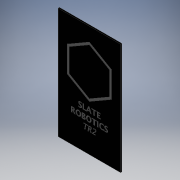
# Autodesk Inventor part: BA03
Saved by Autodesk Inventor 2017 (Build 210142000, 142)
## iProperties
Created: 2018-10-18
Part Number: BA03
Material: ABS Plastic
Document SubType Name: Modeling
Designer: Dell
Density: 1.06 g/cm^3
Appearance: Smooth - Black
Author: Dell
Autodesk Inventor part; units mm, degrees
ref_plane "YZ Plane" through (0, 0, 0) normal (1, 0, 0) x (0, 1, 0)
ref_plane "XZ Plane" through (0, 0, 0) normal (0, 1, 0) x (-1, 0, 0)
ref_plane "XY Plane" through (0, 0, 0) normal (0, 0, 1) x (1, 0, 0)
sketch "Sketch1" plane through (0, 0, 0) normal (0, 0, 1) x (1, 0, 0)
  line L0 (0, 0) -> (303.5592, 0)
  line L1 (303.5592, 0) -> (303.5592, -533.4)
  line L2 (303.5592, -533.4) -> (0, -533.4)
  line L3 (0, -533.4) -> (0, 0)
  line L4 (455.3388, 262.89) -> (303.5592, 0)
  line L5 (303.5592, 0) -> (0, 0)
  line L6 (0, 0) -> (-151.7796, 262.89)
  line L7 (-151.7796, 262.89) -> (0, 525.78)
  line L8 (0, 525.78) -> (303.5592, 525.78)
  line L9 (303.5592, 525.78) -> (455.3388, 262.89)
  point P0 (151.7796, 262.89)
  dimension "d1" = 533.4
  dimension "d76" = 525.78
  constraints: 20 end point, 2 parallel, 1 horizontal, 1 perpendicular, 13 other
  measures "d1" distance of L0.end L1.end
  measures "d76" distance between parallel lines of L4 L7
extrude "Extrusion1" add sketch "Sketch1" along normal blind 6.35 contours L0 L1 L2 L3
sketch "Sketch2" plane through (0, 0, 0) normal (0, 1, 0) x (1, 0, 0)
  line L0 (303.5592, -6.35) -> (0, -6.35) projected
  line L1 (0, -6.35) -> (-3.6662, -6.35)
  line L2 (-3.6662, -6.35) -> (0, 0)
  line L3 (0, 0) -> (0, -6.35) projected
  line L4 (0, 0) -> (0, -6.35) projected
  line L5 (0, -6.35) -> (0, 0)
  line L6 (303.5592, -6.35) -> (307.2254, -6.35)
  line L7 (303.5592, 0) -> (303.5592, -6.35) projected
  line L8 (307.2254, -6.35) -> (303.5592, 0)
  line L9 (303.5592, 0) -> (303.5592, -6.35)
  dimension "d4" = 30
  dimension "d5" = 60
  constraints: 12 end point, 2 collinear, 2 horizontal
  measures "d4" angle of L3 L2
  measures "d5" angle of L6 L8
extrude "Extrusion2" add sketch "Sketch2" against normal blind 533.4
sketch "Sketch6" plane through (0, 0, 6.35) normal (0, 0, 1) x (1, 0, 0)
  line L0 (26.7796, -316.7) -> (276.7796, -316.7) construction
  line L1 (276.7796, -316.7) -> (276.7796, -466.7) construction
  line L2 (276.7796, -466.7) -> (26.7796, -466.7) construction
  line L3 (26.7796, -466.7) -> (26.7796, -316.7) construction
  line L4 (26.7796, -66.7) -> (276.7796, -66.7) construction
  line L5 (276.7796, -66.7) -> (276.7796, -316.7) construction
  line L6 (276.7796, -316.7) -> (26.7796, -316.7) construction
  line L7 (26.7796, -316.7) -> (26.7796, -66.7) construction
  line L8 (276.7796, -466.7) -> (276.7796, -66.7) construction
  line L9 (151.7796, -66.7) -> (260.0328, -129.2)
  line L10 (260.0328, -129.2) -> (260.0328, -254.2)
  line L11 (260.0328, -254.2) -> (151.7796, -316.7)
  line L12 (151.7796, -316.7) -> (43.5264, -254.2)
  line L13 (43.5264, -254.2) -> (43.5264, -129.2)
  line L14 (43.5264, -129.2) -> (151.7796, -66.7)
  line L15 (151.7796, -78.4779) -> (249.8328, -135.089)
  line L16 (249.8328, -135.089) -> (249.8328, -248.311)
  line L17 (249.8328, -248.311) -> (151.7796, -304.9221)
  line L18 (151.7796, -304.9221) -> (53.7264, -248.311)
  line L19 (53.7264, -248.311) -> (53.7264, -135.089)
  line L20 (53.7264, -135.089) -> (151.7796, -78.4779)
  line L21 (151.7796, -83.3854) -> (245.5828, -137.5427) construction
  line L22 (245.5828, -137.5427) -> (245.5828, -245.8573)
  line L23 (245.5828, -245.8573) -> (151.7796, -300.0146)
  line L24 (151.7796, -300.0146) -> (57.9764, -245.8573)
  line L25 (57.9764, -245.8573) -> (57.9764, -137.5427)
  line L26 (57.9764, -137.5427) -> (151.7796, -83.3854) construction
  line L27 (57.9764, -190.0427) -> (97.9764, -166.9487)
  line L28 (97.9764, -166.9487) -> (97.9764, -138.4487)
  line L29 (97.9764, -138.4487) -> (111.9764, -138.4487)
  line L30 (111.9764, -138.4487) -> (111.9764, -158.8658)
  line L31 (111.9764, -158.8658) -> (151.7796, -135.8854)
  line L32 (151.7796, -135.8854) -> (245.5828, -190.0427)
  line L33 (245.5828, -190.0427) -> (245.5828, -137.5427)
  line L34 (245.5828, -137.5427) -> (151.7796, -83.3854)
  line L35 (151.7796, -83.3854) -> (57.9764, -137.5427)
  line L36 (57.9764, -190.0427) -> (57.9764, -137.5427)
  line L37 (57.9764, -245.8573) -> (139.7796, -293.0864)
  line L38 (139.7796, -293.0864) -> (139.7796, -253.0146)
  line L39 (139.7796, -253.0146) -> (163.7796, -253.0146)
  line L40 (163.7796, -253.0146) -> (163.7796, -293.0864)
  line L41 (163.7796, -293.0864) -> (245.5828, -245.8573)
  line L42 (245.5828, -245.8573) -> (245.5828, -205.0427)
  line L43 (245.5828, -205.0427) -> (151.7796, -150.8854)
  line L44 (151.7796, -150.8854) -> (57.9764, -205.0427)
  line L45 (57.9764, -205.0427) -> (57.9764, -245.8573)
  line L46 (125.5296, -179.0146) -> (178.0296, -179.0146) construction
  line L47 (178.0296, -179.0146) -> (178.0296, -230.0146) construction
  line L48 (178.0296, -230.0146) -> (125.5296, -230.0146) construction
  line L49 (125.5296, -230.0146) -> (125.5296, -179.0146) construction
  line L50 (125.5296, -230.0146) -> (149.5296, -230.0146)
  line L51 (149.5296, -230.0146) -> (149.5296, -206.0146)
  line L52 (149.5296, -206.0146) -> (125.5296, -206.0146)
  line L53 (125.5296, -206.0146) -> (125.5296, -230.0146)
  line L54 (125.5296, -179.0146) -> (149.5296, -179.0146)
  line L55 (149.5296, -179.0146) -> (149.5296, -203.0146)
  line L56 (149.5296, -203.0146) -> (125.5296, -203.0146)
  line L57 (125.5296, -203.0146) -> (125.5296, -179.0146)
  line L58 (178.0296, -179.0146) -> (154.0296, -179.0146)
  line L59 (154.0296, -179.0146) -> (154.0296, -203.0146)
  line L60 (154.0296, -203.0146) -> (178.0296, -203.0146)
  line L61 (178.0296, -203.0146) -> (178.0296, -179.0146)
  line L62 (178.0296, -230.0146) -> (154.0296, -230.0146)
  line L63 (154.0296, -230.0146) -> (154.0296, -206.0146)
  line L64 (154.0296, -206.0146) -> (178.0296, -206.0146)
  line L65 (178.0296, -206.0146) -> (178.0296, -230.0146)
  line L66 (-3.6662, 0) -> (307.2254, 0) projected
  line L67 (-3.6662, 0) -> (-3.6662, -533.4) projected
  line L68 (98.5279, -364.3042) -> (98.5279, -360.0196)
  spline S0 degree 2 poles (98.5279, -360.0196) (101.4544, -361.2437) (104.3427, -361.7219) (105.5478, -361.7219) knots 0 0 0 1 2 2 2
  spline S1 degree 2 poles (105.5478, -361.7219) (107.7284, -361.7219) (109.8898, -359.7709) (109.8898, -358.3937) knots 0 0 0 1 2 2 2
  spline S2 degree 2 poles (109.8898, -358.3937) (109.8898, -357.3417) (109.2968, -356.5) knots 0 0 0 1 1 1
  spline S3 degree 2 poles (109.2968, -356.5) (108.6847, -355.6776) (106.332, -354.3577) knots 0 0 0 1 1 1
  line L69 (106.332, -354.3577) -> (104.6488, -353.4205)
  spline S4 degree 2 poles (104.6488, -353.4205) (101.0336, -351.4121) (99.7712, -349.7097) knots 0 0 0 1 1 1
  spline S5 degree 2 poles (99.7712, -349.7097) (98.4705, -348.0073) (98.4705, -345.7694) knots 0 0 0 1 1 1
  spline S6 degree 2 poles (98.4705, -345.7694) (98.4705, -342.9385) (102.7934, -338.9216) (106.8293, -338.9216) knots 0 0 0 1 2 2 2
  spline S7 degree 2 poles (106.8293, -338.9216) (109.8515, -338.9216) (113.6388, -339.7824) knots 0 0 0 1 1 1
  line L70 (113.6388, -339.7824) -> (113.6388, -343.7801)
  spline S8 degree 2 poles (113.6388, -343.7801) (109.7559, -342.3455) (107.4797, -342.3455) knots 0 0 0 1 1 1
  spline S9 degree 2 poles (107.4797, -342.3455) (105.586, -342.3455) (103.6159, -343.9905) (103.6159, -345.1382) knots 0 0 0 1 2 2 2
  spline S10 degree 2 poles (103.6159, -345.1382) (103.6159, -346.018) (104.228, -346.764) knots 0 0 0 1 1 1
  spline S11 degree 2 poles (104.228, -346.764) (104.8018, -347.5291) (107.1545, -348.8489) knots 0 0 0 1 1 1
  line L71 (107.1545, -348.8489) -> (108.9525, -349.8436)
  spline S12 degree 2 poles (108.9525, -349.8436) (113.1033, -352.158) (114.2318, -353.8604) knots 0 0 0 1 1 1
  spline S13 degree 2 poles (114.2318, -353.8604) (115.3603, -355.5819) (115.3603, -357.7242) knots 0 0 0 1 1 1
  spline S14 degree 2 poles (115.3603, -357.7242) (115.3603, -360.8038) (110.674, -365.1458) (105.5669, -365.1458) knots 0 0 0 1 2 2 2
  spline S15 degree 2 poles (105.5669, -365.1458) (102.5447, -365.1458) (98.5279, -364.3042) knots 0 0 0 1 1 1
  line L72 (119.6832, -364.5337) -> (119.6832, -339.5337)
  line L73 (119.6832, -339.5337) -> (124.886, -339.5337)
  line L74 (124.886, -339.5337) -> (124.886, -360.9951)
  line L75 (124.886, -360.9951) -> (136.0375, -360.9951)
  line L76 (136.0375, -360.9951) -> (136.0375, -364.5337)
  line L77 (136.0375, -364.5337) -> (119.6832, -364.5337)
  line L78 (137.0512, -364.5337) -> (146.749, -339.5337)
  line L79 (146.749, -339.5337) -> (151.9709, -339.5337)
  line L80 (151.9709, -339.5337) -> (161.7069, -364.5337)
  line L81 (161.7069, -364.5337) -> (156.3703, -364.5337)
  line L82 (156.3703, -364.5337) -> (153.7689, -357.8581)
  line L83 (153.7689, -357.8581) -> (143.4399, -357.8581)
  line L84 (143.4399, -357.8581) -> (140.8385, -364.5337)
  line L85 (140.8385, -364.5337) -> (137.0512, -364.5337)
  line L86 (144.7215, -354.5299) -> (152.4682, -354.5299)
  line L87 (152.4682, -354.5299) -> (148.6044, -344.5643)
  line L88 (148.6044, -344.5643) -> (144.7215, -354.5299)
  line L89 (171.4621, -364.5337) -> (171.4621, -342.9767)
  line L90 (171.4621, -342.9767) -> (162.5103, -342.9767)
  line L91 (162.5103, -342.9767) -> (162.5103, -339.5337)
  line L92 (162.5103, -339.5337) -> (185.6166, -339.5337)
  line L93 (185.6166, -339.5337) -> (185.6166, -342.9767)
  line L94 (185.6166, -342.9767) -> (176.6648, -342.9767)
  line L95 (176.6648, -342.9767) -> (176.6648, -364.5337)
  line L96 (176.6648, -364.5337) -> (171.4621, -364.5337)
  line L97 (189.0979, -364.5337) -> (189.0979, -339.5337)
  line L98 (189.0979, -339.5337) -> (205.1078, -339.5337)
  line L99 (205.1078, -339.5337) -> (205.1078, -342.9767)
  line L100 (205.1078, -342.9767) -> (194.3007, -342.9767)
  line L101 (194.3007, -342.9767) -> (194.3007, -349.9392)
  line L102 (194.3007, -349.9392) -> (203.2333, -349.9392)
  line L103 (203.2333, -349.9392) -> (203.2333, -353.3822)
  line L104 (203.2333, -353.3822) -> (194.3007, -353.3822)
  line L105 (194.3007, -353.3822) -> (194.3007, -360.9951)
  line L106 (194.3007, -360.9951) -> (205.9112, -360.9951)
  line L107 (205.9112, -360.9951) -> (205.9112, -364.5337)
  line L108 (205.9112, -364.5337) -> (189.0979, -364.5337)
  line L109 (63.7632, -404.4902) -> (63.7632, -379.4902)
  line L110 (63.7632, -379.4902) -> (73.1166, -379.4902)
  spline S16 degree 2 poles (73.1166, -379.4902) (75.9858, -379.4902) (78.9889, -380.9248) (80.7295, -383.8514) (80.7295, -385.6876) knots 0 0 0 1 2 3 3 3
  spline S17 degree 2 poles (80.7295, -385.6876) (80.7295, -387.8873) (78.2046, -391.7894) (75.8902, -392.8223) knots 0 0 0 1 2 2 2
  line L111 (75.8902, -392.8223) -> (84.0577, -404.4902)
  line L112 (84.0577, -404.4902) -> (77.7264, -404.4902)
  line L113 (77.7264, -404.4902) -> (71.5099, -394.276)
  line L114 (71.5099, -394.276) -> (68.6599, -394.276)
  line L115 (68.6599, -394.276) -> (68.6599, -404.4902)
  line L116 (68.6599, -404.4902) -> (63.7632, -404.4902)
  line L117 (68.6599, -390.8521) -> (69.8458, -390.8521)
  spline S18 degree 2 poles (69.8458, -390.8521) (73.0593, -390.8521) (75.5267, -388.0403) (75.5267, -386.2615) knots 0 0 0 1 2 2 2
  spline S19 degree 2 poles (75.5267, -386.2615) (75.5267, -384.7312) (73.5375, -382.9141) (70.477, -382.9141) knots 0 0 0 1 2 2 2
  line L118 (70.477, -382.9141) -> (68.6599, -382.9141)
  line L119 (68.6599, -382.9141) -> (68.6599, -390.8521)
  spline S20 degree 2 poles (98.7479, -405.1023) (94.8458, -405.1023) (89.0692, -401.8697) (86.0662, -395.8253) (86.0662, -391.9807) knots 0 0 0 1 2 3 3 3
  spline S21 degree 2 poles (86.0662, -391.9807) (86.0662, -388.1742) (89.0692, -382.0916) (94.8841, -378.8781) (98.7479, -378.8781) knots 0 0 0 1 2 3 3 3
  spline S22 degree 2 poles (98.7479, -378.8781) (102.5925, -378.8781) (108.4074, -382.0916) (111.4105, -388.1742) (111.4105, -391.9807) knots 0 0 0 1 2 3 3 3
  spline S23 degree 2 poles (111.4105, -391.9807) (111.4105, -395.8253) (108.4074, -401.8697) (102.6499, -405.1023) (98.7479, -405.1023) knots 0 0 0 1 2 3 3 3
  spline S24 degree 2 poles (98.7479, -401.6784) (102.363, -401.6784) (105.8825, -395.7871) (105.8825, -391.9807) knots 0 0 0 1 2 2 2
  spline S25 degree 2 poles (105.8825, -391.9807) (105.8825, -388.1551) (102.3439, -382.302) (98.7479, -382.302) knots 0 0 0 1 2 2 2
  spline S26 degree 2 poles (98.7479, -382.302) (95.1327, -382.302) (91.5941, -388.1551) (91.5941, -391.9807) knots 0 0 0 1 2 2 2
  spline S27 degree 2 poles (91.5941, -391.9807) (91.5941, -395.7871) (95.1136, -401.6784) (98.7479, -401.6784) knots 0 0 0 1 2 2 2
  line L120 (116.0776, -404.4902) -> (116.0776, -379.4902)
  line L121 (116.0776, -379.4902) -> (124.513, -379.4902)
  spline S28 degree 2 poles (124.513, -379.4902) (127.5734, -379.4902) (130.5, -380.8674) (132.1641, -383.5453) (132.1641, -385.0564) knots 0 0 0 1 2 3 3 3
  spline S29 degree 2 poles (132.1641, -385.0564) (132.1641, -386.9309) (129.5627, -390.3739) (126.1962, -391.426) knots 0 0 0 1 2 2 2
  spline S30 degree 2 poles (126.1962, -391.426) (128.8741, -392.0954) (131.705, -394.0465) (133.1779, -396.7626) (133.1779, -398.312) knots 0 0 0 1 2 3 3 3
  spline S31 degree 2 poles (133.1779, -398.312) (133.1779, -399.9952) (131.4564, -402.9217) (128.4342, -404.4902) (125.2972, -404.4902) knots 0 0 0 1 2 3 3 3
  line L122 (125.2972, -404.4902) -> (116.0776, -404.4902)
  line L123 (121.07, -400.9516) -> (122.0646, -400.9516)
  spline S32 degree 2 poles (122.0646, -400.9516) (124.7808, -400.9516) (126.7509, -400.2439) (127.7456, -398.6563) (127.7456, -397.6807) knots 0 0 0 1 2 3 3 3
  spline S33 degree 2 poles (127.7456, -397.6807) (127.7456, -395.8253) (124.4747, -393.2431) (121.969, -393.2431) knots 0 0 0 1 2 2 2
  line L124 (121.969, -393.2431) -> (121.07, -393.2431)
  line L125 (121.07, -393.2431) -> (121.07, -400.9516)
  line L126 (121.07, -389.8957) -> (122.1794, -389.8957)
  spline S34 degree 2 poles (122.1794, -389.8957) (124.5512, -389.8957) (126.8848, -387.543) (126.8848, -385.8598) knots 0 0 0 1 2 2 2
  spline S35 degree 2 poles (126.8848, -385.8598) (126.8848, -384.9608) (126.1962, -383.6409) (124.4556, -382.9141) (122.0072, -382.9141) knots 0 0 0 1 2 3 3 3
  line L127 (122.0072, -382.9141) -> (121.07, -382.9141)
  line L128 (121.07, -382.9141) -> (121.07, -389.8957)
  spline S36 degree 2 poles (148.9965, -405.1023) (145.0945, -405.1023) (139.3179, -401.8697) (136.3148, -395.8253) (136.3148, -391.9807) knots 0 0 0 1 2 3 3 3
  spline S37 degree 2 poles (136.3148, -391.9807) (136.3148, -388.1742) (139.3179, -382.0916) (145.1327, -378.8781) (148.9965, -378.8781) knots 0 0 0 1 2 3 3 3
  spline S38 degree 2 poles (148.9965, -378.8781) (152.8412, -378.8781) (158.6561, -382.0916) (161.6591, -388.1742) (161.6591, -391.9807) knots 0 0 0 1 2 3 3 3
  spline S39 degree 2 poles (161.6591, -391.9807) (161.6591, -395.8253) (158.6561, -401.8697) (152.8986, -405.1023) (148.9965, -405.1023) knots 0 0 0 1 2 3 3 3
  spline S40 degree 2 poles (148.9965, -401.6784) (152.6117, -401.6784) (156.1312, -395.7871) (156.1312, -391.9807) knots 0 0 0 1 2 2 2
  spline S41 degree 2 poles (156.1312, -391.9807) (156.1312, -388.1551) (152.5925, -382.302) (148.9965, -382.302) knots 0 0 0 1 2 2 2
  spline S42 degree 2 poles (148.9965, -382.302) (145.3814, -382.302) (141.8427, -388.1551) (141.8427, -391.9807) knots 0 0 0 1 2 2 2
  spline S43 degree 2 poles (141.8427, -391.9807) (141.8427, -395.7871) (145.3622, -401.6784) (148.9965, -401.6784) knots 0 0 0 1 2 2 2
  line L129 (172.5428, -404.4902) -> (172.5428, -382.9332)
  line L130 (172.5428, -382.9332) -> (163.591, -382.9332)
  line L131 (163.591, -382.9332) -> (163.591, -379.4902)
  line L132 (163.591, -379.4902) -> (186.6974, -379.4902)
  line L133 (186.6974, -379.4902) -> (186.6974, -382.9332)
  line L134 (186.6974, -382.9332) -> (177.7456, -382.9332)
  line L135 (177.7456, -382.9332) -> (177.7456, -404.4902)
  line L136 (177.7456, -404.4902) -> (172.5428, -404.4902)
  line L137 (190.1786, -404.4902) -> (190.1786, -379.4902)
  line L138 (190.1786, -379.4902) -> (195.3814, -379.4902)
  line L139 (195.3814, -379.4902) -> (195.3814, -404.4902)
  line L140 (195.3814, -404.4902) -> (190.1786, -404.4902)
  spline S44 degree 2 poles (221.7586, -403.4956) (220.1136, -404.2224) (217.6844, -404.758) (214.6048, -405.1023) (213.0937, -405.1023) knots 0 0 0 1 2 3 3 3
  spline S45 degree 2 poles (213.0937, -405.1023) (206.5329, -405.1023) (200.0868, -397.719) (200.0868, -391.9807) knots 0 0 0 1 2 2 2
  spline S46 degree 2 poles (200.0868, -391.9807) (200.0868, -386.2423) (206.5137, -378.8781) (213.4189, -378.8781) knots 0 0 0 1 2 2 2
  spline S47 degree 2 poles (213.4189, -378.8781) (217.4931, -378.8781) (221.529, -379.8345) knots 0 0 0 1 1 1
  line L141 (221.529, -379.8345) -> (221.529, -383.9087)
  spline S48 degree 2 poles (221.529, -383.9087) (219.578, -383.2393) (217.1105, -382.608) (214.9108, -382.302) (213.8014, -382.302) knots 0 0 0 1 2 3 3 3
  spline S49 degree 2 poles (213.8014, -382.302) (209.4977, -382.302) (205.6147, -387.8299) (205.6147, -391.9233) knots 0 0 0 1 2 2 2
  spline S50 degree 2 poles (205.6147, -391.9233) (205.6147, -396.2079) (210.0141, -401.5063) (214.3753, -401.5063) knots 0 0 0 1 2 2 2
  spline S51 degree 2 poles (214.3753, -401.5063) (218.0095, -401.5063) (221.7586, -399.67) knots 0 0 0 1 1 1
  line L142 (221.7586, -399.67) -> (221.7586, -403.4956)
  line L143 (224.8764, -404.2607) -> (224.8764, -399.9761)
  spline S52 degree 2 poles (224.8764, -399.9761) (227.803, -401.2002) (230.6912, -401.6784) (231.8963, -401.6784) knots 0 0 0 1 2 2 2
  spline S53 degree 2 poles (231.8963, -401.6784) (234.0769, -401.6784) (236.2383, -399.7274) (236.2383, -398.3502) knots 0 0 0 1 2 2 2
  spline S54 degree 2 poles (236.2383, -398.3502) (236.2383, -397.2982) (235.6453, -396.4566) knots 0 0 0 1 1 1
  spline S55 degree 2 poles (235.6453, -396.4566) (235.0333, -395.6341) (232.6805, -394.3142) knots 0 0 0 1 1 1
  line L144 (232.6805, -394.3142) -> (230.9973, -393.377)
  spline S56 degree 2 poles (230.9973, -393.377) (227.3821, -391.3686) (226.1197, -389.6662) knots 0 0 0 1 1 1
  spline S57 degree 2 poles (226.1197, -389.6662) (224.819, -387.9638) (224.819, -385.7259) knots 0 0 0 1 1 1
  spline S58 degree 2 poles (224.819, -385.7259) (224.819, -382.895) (229.1419, -378.8781) (233.1779, -378.8781) knots 0 0 0 1 2 2 2
  spline S59 degree 2 poles (233.1779, -378.8781) (236.2, -378.8781) (239.9873, -379.7389) knots 0 0 0 1 1 1
  line L145 (239.9873, -379.7389) -> (239.9873, -383.7366)
  spline S60 degree 2 poles (239.9873, -383.7366) (236.1044, -382.302) (233.8282, -382.302) knots 0 0 0 1 1 1
  spline S61 degree 2 poles (233.8282, -382.302) (231.9346, -382.302) (229.9644, -383.947) (229.9644, -385.0947) knots 0 0 0 1 2 2 2
  spline S62 degree 2 poles (229.9644, -385.0947) (229.9644, -385.9745) (230.5765, -386.7205) knots 0 0 0 1 1 1
  spline S63 degree 2 poles (230.5765, -386.7205) (231.1503, -387.4856) (233.503, -388.8054) knots 0 0 0 1 1 1
  line L146 (233.503, -388.8054) -> (235.301, -389.8001)
  spline S64 degree 2 poles (235.301, -389.8001) (239.4518, -392.1146) (240.5803, -393.8169) knots 0 0 0 1 1 1
  spline S65 degree 2 poles (240.5803, -393.8169) (241.7088, -395.5384) (241.7088, -397.6807) knots 0 0 0 1 1 1
  spline S66 degree 2 poles (241.7088, -397.6807) (241.7088, -400.7603) (237.0225, -405.1023) (231.9154, -405.1023) knots 0 0 0 1 2 2 2
  spline S67 degree 2 poles (231.9154, -405.1023) (228.8932, -405.1023) (224.8764, -404.2607) knots 0 0 0 1 1 1
  line L147 (128.1258, -444.4784) -> (132.5873, -422.1322)
  line L148 (132.5873, -422.1322) -> (123.7027, -422.1322)
  line L149 (123.7027, -422.1322) -> (124.2219, -419.4784)
  line L150 (124.2219, -419.4784) -> (145.5104, -419.4784)
  line L151 (145.5104, -419.4784) -> (144.9719, -422.1322)
  line L152 (144.9719, -422.1322) -> (136.1065, -422.1322)
  line L153 (136.1065, -422.1322) -> (131.6642, -444.4784)
  line L154 (131.6642, -444.4784) -> (128.1258, -444.4784)
  line L155 (143.9142, -444.4784) -> (148.895, -419.4784)
  line L156 (148.895, -419.4784) -> (156.4335, -419.4784)
  spline S68 degree 2 poles (156.4335, -419.4784) (158.4142, -419.4784) (161.1258, -420.1515) (162.9142, -422.5745) (162.9142, -424.3245) knots 0 0 0 1 2 3 3 3
  spline S69 degree 2 poles (162.9142, -424.3245) (162.9142, -426.863) (159.2988, -431.363) (156.2219, -432.5361) knots 0 0 0 1 2 2 2
  line L157 (156.2219, -432.5361) -> (162.1642, -444.4784)
  line L158 (162.1642, -444.4784) -> (158.2412, -444.4784)
  line L159 (158.2412, -444.4784) -> (152.9912, -433.4207)
  line L160 (152.9912, -433.4207) -> (149.645, -433.4207)
  line L161 (149.645, -433.4207) -> (147.4527, -444.4784)
  line L162 (147.4527, -444.4784) -> (143.9142, -444.4784)
  line L163 (150.1642, -430.8053) -> (152.1258, -430.8053)
  spline S70 degree 2 poles (152.1258, -430.8053) (154.2219, -430.8053) (157.3181, -429.2284) (159.145, -426.2284) (159.145, -424.7284) knots 0 0 0 1 2 3 3 3
  spline S71 degree 2 poles (159.145, -424.7284) (159.145, -423.4399) (157.1835, -422.1322) (154.145, -422.1322) knots 0 0 0 1 2 2 2
  line L164 (154.145, -422.1322) -> (151.895, -422.1322)
  line L165 (151.895, -422.1322) -> (150.1642, -430.8053)
  line L166 (165.8565, -444.4784) -> (166.395, -441.7861)
  spline S72 degree 2 poles (166.395, -441.7861) (167.5296, -439.7091) (170.7412, -436.4015) (173.0873, -434.5938) knots 0 0 0 1 2 2 2
  line L167 (173.0873, -434.5938) -> (175.1835, -432.9976)
  spline S73 degree 2 poles (175.1835, -432.9976) (178.1642, -430.7091) (179.7604, -428.7668) knots 0 0 0 1 1 1
  spline S74 degree 2 poles (179.7604, -428.7668) (180.5681, -427.7861) (181.3758, -425.8438) (181.3758, -424.8822) knots 0 0 0 1 2 2 2
  spline S75 degree 2 poles (181.3758, -424.8822) (181.3758, -423.3053) (179.2027, -421.363) (177.0681, -421.363) knots 0 0 0 1 2 2 2
  spline S76 degree 2 poles (177.0681, -421.363) (174.0681, -421.363) (170.4719, -423.4015) knots 0 0 0 1 1 1
  line L168 (170.4719, -423.4015) -> (171.0681, -420.4207)
  spline S77 degree 2 poles (171.0681, -420.4207) (171.645, -420.2091) (171.9142, -420.0745) knots 0 0 0 1 1 1
  spline S78 degree 2 poles (171.9142, -420.0745) (175.2027, -418.863) (177.9142, -418.863) knots 0 0 0 1 1 1
  spline S79 degree 2 poles (177.9142, -418.863) (181.1065, -418.863) (184.9142, -421.6515) (184.9142, -424.4784) knots 0 0 0 1 2 2 2
  spline S80 degree 2 poles (184.9142, -424.4784) (184.9142, -425.9784) (184.3758, -427.3053) knots 0 0 0 1 1 1
  spline S81 degree 2 poles (184.3758, -427.3053) (183.5681, -429.3438) (180.6258, -432.1899) (177.9142, -434.1707) knots 0 0 0 1 2 2 2
  line L169 (177.9142, -434.1707) -> (175.8181, -435.6899)
  spline S82 degree 2 poles (175.8181, -435.6899) (173.9335, -437.0745) (172.5296, -438.3822) (171.8758, -439.1707) knots 0 0 0 1 2 2 2
  spline S83 degree 2 poles (171.8758, -439.1707) (171.4912, -439.6707) (170.7796, -440.6322) (170.3758, -441.5745) knots 0 0 0 1 2 2 2
  line L170 (170.3758, -441.5745) -> (181.3373, -441.5745)
  line L171 (181.3373, -441.5745) -> (180.7412, -444.4784)
  line L172 (180.7412, -444.4784) -> (165.8565, -444.4784)
  point P0 (0, 0)
  point P1 (151.7796, -191.7)
  point P2 (151.7796, -253.0146)
  point P3 (151.7796, -179.0146)
  point P4 (276.7796, -266.7)
  point P5 (-3.6662, -266.7)
  point P6 (151.7796, 0)
  dimension "d27" = 250
  dimension "d28" = 10.2
  dimension "d29" = 4.25
  dimension "d30" = 52.5
  dimension "d31" = 40
  dimension "d32" = 14
  dimension "d33" = 28.5
  dimension "d34" = 15
  dimension "d35" = 24
  dimension "d36" = 47
  dimension "d37" = 23
  dimension "d38" = 51
  dimension "d39" = 52.5
  dimension "d40" = 24
  dimension "d41" = 24
  dimension "d42" = 24
  dimension "d43" = 24
  dimension "d44" = 24
  dimension "d45" = 24
  dimension "d46" = 24
  dimension "d47" = 24
  dimension "d66" = 150
  constraints: 116 end point, 15 parallel, 9 perpendicular, 9 point on line, 8 midpoint, 6 vertical alignment, 5 horizontal, 4 collinear, 2 coincident, 2 vertical, 1 horizontal alignment, 26 other
  measures "d27" distance of L7.end L5.start
  measures "d28" distance between parallel lines of L14 L20
  measures "d29" distance between parallel lines of L20 L26
  measures "d30" distance of L27.start L25.end
  measures "d31" distance between parallel lines of L25 L28
  measures "d32" distance of L28.end L29.end
  measures "d33" distance of L27.end L28.end
  measures "d34" distance of L32.start L43.end
  measures "d35" distance between parallel lines of L40 L38
  measures "d36" distance from line of L24.start L39
  measures "d37" distance between parallel lines of L39 L48
  measures "d38" distance of L50.start L54.start
  measures "d39" distance of L54.start L61.end
  measures "d40" distance of L52.end L52.start
  measures "d41" distance of L52.start L51.start
  measures "d42" distance of L55.end L57.start
  measures "d43" distance of L55.start L55.end
  measures "d44" distance of L61.start L59.end
  measures "d45" distance of L59.end L59.start
  measures "d46" distance of L64.start L64.end
  measures "d47" distance of L63.start L64.start
  measures "d66" distance between parallel lines of L2 L6
extrude "Extrusion5" cut sketch "Sketch6" against normal blind 2 contours L9 L10 L11 L12 L13 L14 | L22 L32 L31 L30 L29 L28 L27 L25 L35 L34 | L22 L43 L44 L25 L27 L28 L29 L30 L31 L32 | L22 L23 L40 L39 L38 L24 L25 L44 L43 | L23 L24 L38 L39 L40 | L53 L52 L51 L50 | L54 L55 L56 L57 | L61 L60 L59 L58 | L62 L63 L64 L65 | L68 S0 S1 S2 S3 L69 S4 S5 S6 S7 L70 S8 S9 S10 S11 L71 S12 S13 S14 S15 | L72 L73 L74 L75 L76 L77 | L78 L79 L80 L81 L82 L83 L84 L85 | L89 L90 L91 L92 L93 L94 L95 L96 | L97 L98 L99 L100 L101 L102 L103 L104 L105 L106 L107 L108 | L109 L110 S16 S17 L111 L112 L113 L114 L115 L116 | S20 S21 S22 S23 | L120 L121 S28 S29 S30 S31 L122 | S36 S37 S38 S39 | L129 L130 L131 L132 L133 L134 L135 L136 | L137 L138 L139 L140 | S44 S45 S46 S47 L141 S48 S49 S50 S51 L142 | L143 S52 S53 S54 S55 L144 S56 S57 S58 S59 L145 S60 S61 S62 S63 L146 S64 S65 S66 S67 | L147 L148 L149 L150 L151 L152 L153 L154 | L155 L156 S68 S69 L157 L158 L159 L160 L161 L162 | L166 S72 L167 S73 S74 S75 S76 L168 S77 S78 S79 S80 S81 L169 S82 S83 L170 L171 L172
extrude "Extrusion6" add sketch "Sketch6" against normal blind 2 contours L22 L32 L31 L30 L29 L28 L27 L25 L35 L34 | L22 L43 L44 L25 L27 L28 L29 L30 L31 L32 | L22 L23 L40 L39 L38 L24 L25 L44 L43 | L23 L24 L38 L39 L40 | L53 L52 L51 L50 | L54 L55 L56 L57 | L61 L60 L59 L58 | L62 L63 L64 L65
sketch "Sketch7" plane through (0, 0, 0) normal (0, 1, 0) x (1, 0, 0)
  line L0 (-3.6662, -6.35) -> (0, 0) projected
  line L1 (0, 0) -> (-3.6662, 0)
  line L2 (-3.6662, 0) -> (-3.6662, -6.35)
  line L3 (-3.6662, -6.35) -> (0, -6.35)
  line L4 (0, -6.35) -> (0, 0)
  line L5 (303.5592, 0) -> (0, 0) projected
  line L6 (303.5592, 0) -> (307.2254, -6.35) projected
  line L7 (303.5592, 0) -> (307.2254, 0)
  line L8 (307.2254, 0) -> (307.2254, -6.35)
  line L9 (307.2254, -6.35) -> (303.5592, -6.35)
  line L10 (303.5592, -6.35) -> (303.5592, 0)
  constraints: 16 end point, 4 parallel, 2 horizontal, 2 perpendicular
extrude "Extrusion7" cut sketch "Sketch7" against normal through all
sketch "Sketch8" plane through (0, 0, 6.35) normal (0, 0, 1) x (1, 0, 0)
  line L0 (303.5592, -533.4) -> (0, -533.4) projected
  line L1 (0, -533.4) -> (303.5592, -533.4)
  line L2 (303.5592, -533.4) -> (303.5592, -539.75)
  line L3 (303.5592, -539.75) -> (0, -539.75)
  line L4 (0, -539.75) -> (0, -533.4)
  point P0 (0, 0)
  dimension "d79" = 6.35
  constraints: 8 end point, 2 parallel, 1 coincident, 1 horizontal, 1 perpendicular
  measures "d79" distance of L3.end L0.end
extrude "Extrusion8" add sketch "Sketch8" against normal blind 6.35
body "Solid1"
